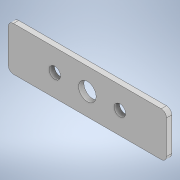
# Autodesk Inventor part: de giu truc Z
Saved by Autodesk Inventor 2020 (Build 240168000, 168)
## iProperties
Created: 2021-05-26
Part Number: de giu truc Z
Material: Generic
Document SubType Name: Modeling
Designer: admin
Density: 1 g/cm^3
Appearance: Default
Author: admin
Autodesk Inventor part; units mm, degrees
ref_plane "YZ Plane" through (0, 0, 0) normal (1, 0, 0) x (0, 1, 0)
ref_plane "XZ Plane" through (0, 0, 0) normal (0, 1, 0) x (-1, 0, 0)
ref_plane "XY Plane" through (0, 0, 0) normal (0, 0, 1) x (1, 0, 0)
sketch "Sketch1" plane through (0, 0, 0) normal (0, 0, 1) x (1, 0, 0)
  line L0 (-45, -12.5) -> (45, -12.5)
  line L1 (45, -12.5) -> (45, 12.5)
  line L2 (45, 12.5) -> (-45, 12.5)
  line L3 (-45, 12.5) -> (-45, -12.5)
  line L4 (-45, -12.5) -> (45, 12.5) construction
  line L5 (45, -12.5) -> (-45, 12.5) construction
  circle A0 centre (-18.5, 0) radius 3.25
  circle A1 centre (18.5, 0) radius 3.25
  point P0 (0, 0)
  dimension "d0" = 90
  dimension "d1" = 25
  dimension "d2" = 37
  dimension "d3" = 18.5
  dimension "d4" = 6.5
  dimension "d5" = 6.5
  dimension "d8" = 12.5
  dimension "d9" = 12.5
  constraints: 12 end point, 2 centre point, 2 midpoint, 2 parallel, 1 horizontal, 1 perpendicular
  measures "d0" distance of L2.end L1.end
  measures "d1" distance of L1.end L0.end
  measures "d2" distance of A1.centre A0.centre
  measures "d3" distance of point (0, 0) A0.centre
  measures "d4" diameter of A0
  measures "d5" diameter of A1
  measures "d8" distance from line of L2 A0.centre
  measures "d9" distance from line of L2 A1.centre
extrude "Extrusion1" add sketch "Sketch1" along normal blind 3
fillet "Fillet1" radius 3 4 edges at (45, 12.5, 1.5) (45, -12.5, 1.5) (-45, 12.5, 1.5) (-45, -12.5, 1.5)
sketch "Sketch2" plane through (0, 0, 3) normal (0, 0, 1) x (1, 0, 0)
  circle A0 centre (0, 0) radius 5
  dimension "d11" = 10
  constraints: 1 centre point, 1 coincident
  measures "d11" diameter of A0
extrude "Extrusion2" cut sketch "Sketch2" against normal blind 10
body "Solid1"
